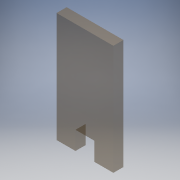
# Autodesk Inventor part: LimitSwitchMount
Saved by Autodesk Inventor 2019 (Build 230136000, 136)
## iProperties
Created: 2019-01-18
Part Number: LimitSwitchMount
Material: Polycarbonate, Smoke
Document SubType Name: Modeling
Designer: nxgam
Density: 1.2 g/cm^3
Appearance: Polycarbonate - Smoked
Author: nxgam
Autodesk Inventor part; units mm, degrees
ref_plane "YZ Plane" through (0, 0, 0) normal (1, 0, 0) x (0, 1, 0)
ref_plane "XZ Plane" through (0, 0, 0) normal (0, 1, 0) x (-1, 0, 0)
ref_plane "XY Plane" through (0, 0, 0) normal (0, 0, 1) x (1, 0, 0)
sketch "Sketch1" plane through (0, 0, 0) normal (0, 0, 1) x (1, 0, 0)
  line L0 (0, 0) -> (15.748, 0)
  line L1 (15.748, 0) -> (15.748, 25.4)
  line L2 (15.748, 25.4) -> (0, 25.4)
  line L3 (0, 25.4) -> (0, 0)
  line L4 (0, 0) -> (5.2493, 0)
  line L5 (5.2493, 0) -> (5.2493, -5.08)
  line L6 (5.2493, -5.08) -> (0, -5.08)
  line L7 (0, -5.08) -> (0, 0)
  line L8 (10.4987, 0) -> (15.748, 0)
  line L9 (15.748, 0) -> (15.748, -5.08)
  line L10 (15.748, -5.08) -> (10.4987, -5.08)
  line L11 (10.4987, -5.08) -> (10.4987, 0)
  dimension "d0" = 25.4
  dimension "d1" = 15.748
  dimension "d2" = 5.2493
  dimension "d3" = 5.08
  dimension "d4" = 0
  dimension "d5" = 5.2493
  constraints: 24 end point, 6 parallel, 3 horizontal, 3 perpendicular, 2 collinear, 2 point on line
  measures "d0" distance of L2.end L0.start
  measures "d1" distance of L0.start L0.end
  measures "d2" distance of L5.end L6.end
  measures "d3" distance of L6.end L4.start
  measures "d4" distance between parallel lines of L3 L7
  measures "d5" distance of L9.end L10.end
extrude "Extrusion1" add sketch "Sketch1" along normal blind 2.794
sketch "Sketch2" plane through (0, 0, 2.794) normal (0, 0, 1) x (1, 0, 0)
  circle A0 centre (3.048, 22.352) radius 1.651 projected
  circle A1 centre (12.7, 3.048) radius 1.651 projected
  line L0 (10.4987, 0) -> (10.4987, -5.08) projected
  line L1 (10.4987, -5.08) -> (15.748, -5.08) projected
  line L2 (15.748, -5.08) -> (15.748, 25.4) projected
  line L3 (15.748, 25.4) -> (0, 25.4) projected
  line L4 (0, 25.4) -> (0, -5.08) projected
  line L5 (0, -5.08) -> (5.2493, -5.08) projected
  line L6 (5.2493, -5.08) -> (5.2493, 0) projected
  line L7 (5.2493, 0) -> (10.4987, 0) projected
  line L8 (5.2493, 0) -> (10.4987, 0) construction
  line L9 (7.874, 0) -> (7.874, 25.4) construction
  line L10 (7.874, 12.7) -> (15.748, 12.7) construction
  circle A2 centre (12.7, 22.352) radius 1.651
  circle A3 centre (3.048, 3.048) radius 1.651
  point P0 (0, 0)
  constraints: 4 end point, 3 midpoint, 2 centre point, 2 symmetric about line, 1 perpendicular, 1 point on line, 2 other
extrude "Extrusion2" cut sketch "Sketch2" against normal blind 25.4 contours A0 | A1 | A2 | A3
sketch "Sketch3" plane through (0, 0, 2.794) normal (0, 0, 1) x (1, 0, 0)
  circle A0 centre (12.7, 22.352) radius 1.651 projected
  circle A1 centre (3.048, 22.352) radius 1.651 projected
  circle A2 centre (12.7, 3.048) radius 1.651 projected
  circle A3 centre (3.048, 3.048) radius 1.651 projected
  line L0 (10.4987, 0) -> (10.4987, -5.08) projected
  line L1 (10.4987, -5.08) -> (15.748, -5.08) projected
  line L2 (15.748, -5.08) -> (15.748, 25.4) projected
  line L3 (15.748, 25.4) -> (0, 25.4) projected
  line L4 (0, 25.4) -> (0, -5.08) projected
  line L5 (0, -5.08) -> (5.2493, -5.08) projected
  line L6 (5.2493, -5.08) -> (5.2493, 0) projected
  line L7 (5.2493, 0) -> (10.4987, 0) projected
  line L8 (0, 0) -> (-3.81, 0)
  line L9 (-3.81, 0) -> (-3.81, 26.035)
  line L10 (-0.635, 29.21) -> (16.383, 29.21)
  line L11 (19.558, 26.035) -> (19.558, 0)
  line L12 (19.558, 0) -> (15.748, 0)
  arc A4 (-0.635, 29.21) -> (-3.81, 26.035) centre (-0.635, 26.035) ccw
  arc A5 (19.558, 26.035) -> (16.383, 29.21) centre (16.383, 26.035) ccw
  line L13 (0, 0) -> (0, 25.4)
  line L14 (15.748, 25.4) -> (0, 25.4) projected
  line L15 (0, 25.4) -> (15.748, 25.4)
  line L16 (15.748, 25.4) -> (15.748, 0)
  dimension "d10" = 3.81
  dimension "d11" = 3.81
  dimension "d12" = 3.81
  dimension "d13" = 3.175
  constraints: 16 end point, 4 perpendicular, 4 point on circle, 4 tangent, 3 point on line, 2 centre point, 2 horizontal, 1 collinear, 1 equal radius
  measures "d10" distance between parallel lines of L9 L4
  measures "d11" distance between parallel lines of L10 L3
  measures "d12" distance between parallel lines of L11 L2
  measures "d13" radius of A4
extrude "Extrusion3" add sketch "Sketch3" against normal blind 2.794 contours L2 L3 L4 L8 L9 A4 L10 A5 L11 L12
equation "\"d2\" = 0.333333 * d1"
equation "\"d5\" = d2"
equation "\"d11\" = d10"
equation "\"d12\" = d11"
body "Solid1"
